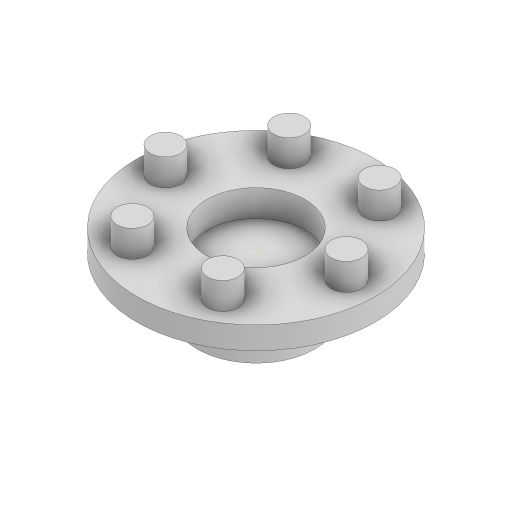
# Autodesk Inventor part: Dysk_wy
Saved by Autodesk Inventor 2024 (Build 280153000, 153)
## iProperties
Created: 2024-12-22
Part Number: Dysk_wy
Material: Ogólny
Document SubType Name: Modeling
Designer: Wicek
Density: 1 g/cm^3
Appearance: Domyślna
Author: Wicek
Autodesk Inventor part; units mm, degrees
ref_plane "YZ Plane" through (0, 0, 0) normal (1, 0, 0) x (0, 1, 0)
ref_plane "XZ Plane" through (0, 0, 0) normal (0, 1, 0) x (-1, 0, 0)
ref_plane "XY Plane" through (0, 0, 0) normal (0, 0, 1) x (1, 0, 0)
sketch "Szkic1" plane through (0, 0, 0) normal (0, 1, 0) x (-1, 0, 0)
  circle A0 centre (0, 0) radius 26.738
  dimension "d0" = 26.738
  constraints: 1 centre point, 1 coincident
  measures "d0" radius of A0
extrude "Wyciągnięcie proste1" add sketch "Szkic1" along normal blind 5
sketch "Szkic2" plane through (0, 5, 0) normal (0, 1, 0) x (1, 0, 0)
  circle A0 centre (-1.4324, 0) radius 18.869 construction
  circle A1 centre (-20.3014, 0) radius 3.4345
  point P0 (0, 0)
  dimension "d5" = 3.4345
  dimension "d6" = 18.869
  constraints: 1 centre point, 1 coincident, 1 horizontal alignment, 2 other
  measures "d5" radius of A1
  measures "d6" distance of A1.centre point (-1.432, 0)
extrude "Wyciągnięcie proste2" add sketch "Szkic2" along normal blind 6
pattern_circular "Szyk kołowy1" count 6 over 360 about axis through (0, 0, 0) along (0, 1, 0) of "Wyciągnięcie proste2"
sketch "Szkic5" plane through (0, 0, 0) normal (0, -1, 0) x (1, 0, 0)
  point P0 (0, 0)
sketch "Szkic6" plane through (0, 0, 0) normal (0, -1, 0) x (1, 0, 0)
  circle A0 centre (0, 0) radius 13.2
  dimension "d17" = 13.2
  constraints: 1 centre point, 1 coincident
  measures "d17" radius of A0
extrude "Wyciągnięcie proste5" add sketch "Szkic6" along normal blind 12
sketch "Szkic7" plane through (0, 5, 0) normal (0, 1, 0) x (1, 0, 0)
  circle A0 centre (0, 0) radius 11
  dimension "d20" = 11
  constraints: 1 centre point, 1 coincident
  measures "d20" radius of A0
extrude "Wyciągnięcie proste6" cut sketch "Szkic7" against normal blind 6
equation "\"d0\" = R"
equation "\"d3\" = h2"
equation "\"d5\" = dwr1"
equation "\"d6\" = dwr2"
equation "\"d17\" = 1.2 * Lrz"
equation "\"d18\" = h2 + Lh"
equation "\"d20\" = Lrz"
equation "\"silnik_rw\" = 2.5"
equation "\"silnik_d_srub\" = 31"
equation "\"silnik_r_wypust\" = Lrz"
equation "\"Lrz\" = 11"
equation "\"Lh\" = 7"
equation "\"Lrw\" = 4"
equation "\"h2\" = 5"
equation "\"h1\" = 2"
equation "\"Rr\" = 2"
equation "\"E1\" = 1"
equation "\"dwr\" = R"
equation "\"dwr2\" = 0.5 * Lrz + 0.5 * R"
equation "\"dwr1\" = -0.25 * Rr + 0.25 * R - 0.25 * Lrz"
equation "\"R1\" = 5"
equation "\"korpus_rw\" = 36.5"
equation "\"R\" = 26.73803"
